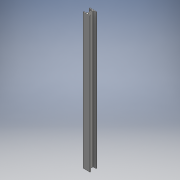
# Autodesk Inventor part: Support beam
Saved by Autodesk Inventor 2016 SP1 (Build 200210100, 210)
## iProperties
Created: 2016-02-19
Part Number: Support beam
Material: Generic
Document SubType Name: Modeling
Designer: Tore Den Store
Density: 1 g/cm^3
Appearance: Default
Author: Tore Den Store
Autodesk Inventor part; units mm, degrees
ref_plane "YZ Plane" through (0, 0, 0) normal (1, 0, 0) x (0, 1, 0)
ref_plane "XZ Plane" through (0, 0, 0) normal (0, 1, 0) x (-1, 0, 0)
ref_plane "XY Plane" through (0, 0, 0) normal (0, 0, 1) x (1, 0, 0)
sketch "Sketch1" plane through (0, 0, 0) normal (0, 0, 1) x (1, 0, 0)
  line L0 (0, 0) -> (100, 0)
  line L1 (100, 0) -> (100, -10)
  line L2 (100, -10) -> (55, -10)
  line L3 (55, -10) -> (55, -90)
  line L4 (55, -90) -> (100, -90)
  line L5 (100, -90) -> (100, -100)
  line L6 (100, -100) -> (0, -100)
  line L7 (0, -100) -> (0, -90)
  line L8 (0, -90) -> (45, -90)
  line L9 (45, -90) -> (45, -10)
  line L10 (45, -10) -> (0, -10)
  line L11 (0, 0) -> (0, -10)
  dimension "d0" = 100
  dimension "d1" = 10
  dimension "d2" = 45
  dimension "d3" = 80
  dimension "d4" = 10
  dimension "d5" = 100
  dimension "d6" = 45
  constraints: 24 end point, 7 perpendicular, 7 point on line, 1 coincident, 1 horizontal
  measures "d0" distance of L0.start L0.end
  measures "d1" distance of L0.end L1.end
  measures "d2" distance of L1.end L2.end
  measures "d3" distance of L2.end L3.end
  measures "d4" distance of L4.end L5.end
  measures "d5" distance of L5.end L6.end
  measures "d6" distance of L7.end L8.end
extrude "Extrusion1" add sketch "Sketch1" along normal blind 2000
fillet "Fillet1" radius 10 4 edges at (55, -10, 1000) (55, -90, 1000) (45, -90, 1000) (45, -10, 1000)
body "Solid1"
